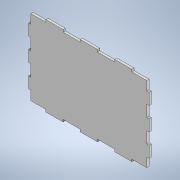
# Autodesk Inventor part: back
Saved by Autodesk Inventor 2020 (Build 240168000, 168)
## iProperties
Created: 2020-02-22
Part Number: back
Material: Generic
Document SubType Name: Modeling
Designer: udvarhelyi
Density: 1 g/cm^3
Appearance: Default
Author: udvarhelyi
Autodesk Inventor part; units mm, degrees
ref_plane "YZ Plane" through (0, 0, 0) normal (1, 0, 0) x (0, 1, 0)
ref_plane "XZ Plane" through (0, 0, 0) normal (0, 1, 0) x (-1, 0, 0)
ref_plane "XY Plane" through (0, 0, 0) normal (0, 0, 1) x (1, 0, 0)
sketch "Sketch1" plane through (0, 0, 0) normal (0, 0, 1) x (1, 0, 0)
  line L0 (-79, 15) -> (-76, 15)
  line L1 (-76, 30) -> (-79, 30)
  line L2 (-79, 45) -> (-76, 45)
  line L3 (-76, 60) -> (-79, 60)
  line L4 (-79, 75) -> (-76, 75)
  line L5 (-76, 90) -> (-79, 90)
  line L6 (76, 15) -> (79, 15)
  line L7 (76, 30) -> (79, 30)
  line L8 (79, 45) -> (76, 45)
  line L9 (76, 60) -> (79, 60)
  line L10 (79, 75) -> (76, 75)
  line L11 (79, 90) -> (76, 90)
  line L12 (-56.4286, 0) -> (-56.4286, 3)
  line L13 (-33.8571, 3) -> (-33.8571, 0)
  line L14 (-11.2857, 0) -> (-11.2857, 3)
  line L15 (11.2857, 0) -> (11.2857, 3)
  line L16 (33.8571, 0) -> (33.8571, 3)
  line L17 (56.4286, 0) -> (56.4286, 3)
  line L18 (-56.4286, 102) -> (-56.4286, 105)
  line L19 (-33.8571, 102) -> (-33.8571, 105)
  line L20 (-11.2857, 102) -> (-11.2857, 105)
  line L21 (11.2857, 102) -> (11.2857, 105)
  line L22 (33.8571, 102) -> (33.8571, 105)
  line L23 (56.4286, 102) -> (56.4286, 105)
  line L24 (-56.4286, 3) -> (-76, 3)
  line L25 (-76, 3) -> (-76, 15)
  line L26 (-76, 30) -> (-76, 45)
  line L27 (-76, 60) -> (-76, 75)
  line L28 (-76, 90) -> (-76, 102)
  line L29 (-76, 102) -> (-56.4286, 102)
  line L30 (-33.8571, 102) -> (-11.2857, 102)
  line L31 (11.2857, 102) -> (33.8571, 102)
  line L32 (56.4286, 102) -> (76, 102)
  line L33 (-11.2857, 3) -> (-33.8571, 3)
  line L34 (76, 3) -> (56.4286, 3)
  line L35 (33.8571, 3) -> (11.2857, 3)
  line L36 (-79, 75) -> (-79, 90)
  line L37 (-79, 15) -> (-79, 30)
  line L38 (-79, 45) -> (-79, 60)
  line L39 (-33.8571, 0) -> (-56.4286, 0)
  line L40 (56.4286, 0) -> (33.8571, 0)
  line L41 (11.2857, 0) -> (-11.2857, 0)
  line L42 (-56.4286, 105) -> (-33.8571, 105)
  line L43 (-11.2857, 105) -> (11.2857, 105)
  line L44 (33.8571, 105) -> (56.4286, 105)
  line L45 (79, 30) -> (79, 15)
  line L46 (79, 90) -> (79, 75)
  line L47 (79, 60) -> (79, 45)
  line L48 (76, 102) -> (76, 90)
  line L49 (76, 75) -> (76, 60)
  line L50 (76, 45) -> (76, 30)
  line L51 (76, 15) -> (76, 3)
  point P0 (0, 0)
  dimension "d1" = 158
  dimension "d5" = 22.5714
  dimension "d6" = 79
  dimension "d7" = 45.1429
  dimension "d8" = 67.7143
  dimension "d9" = 90.2857
  dimension "d10" = 112.8571
  dimension "d11" = 135.4286
  dimension "d12" = 105
  dimension "d13" = 15
  dimension "d14" = 0
  dimension "d15" = 3
  dimension "d16" = 30
  dimension "d17" = 45
  dimension "d18" = 60
  dimension "d19" = 75
  dimension "d20" = 90
  dimension "d21" = 99
  dimension "d22" = 3
  dimension "d23" = 3
  constraints: 104 end point, 79 perpendicular, 53 parallel, 21 collinear, 18 point on line, 3 horizontal
  measures "d1" distance of L5.end L11.start
  measures "d5" distance from line of L17.start L45
  measures "d6" distance from line of L46 point (0, 0)
  measures "d7" distance from line of L45 L16.start
  measures "d8" distance from line of L45 L15.end
  measures "d9" distance from line of L45 L14.start
  measures "d10" distance from line of L45 L13.end
  measures "d11" distance from line of L45 L12.start
  measures "d12" distance from line of L43 point (0, 0)
  measures "d13" distance from line of L0.start L39
  measures "d14" distance from line of point (0, 0) L39
  measures "d15" distance of L12.start L12.end
  measures "d16" distance from line of L39 L1.end
  measures "d17" distance from line of L39 L2.end
  measures "d18" distance from line of L39 L3.end
  measures "d19" distance from line of L39 L4.end
  measures "d20" distance from line of L39 L5.end
  measures "d21" distance between parallel lines of L24 L29
  measures "d22" distance of L11.start L11.end
  measures "d23" distance of L5.start L5.end
extrude "Extrusion1" add sketch "Sketch1" along normal blind 3
equation "\"d1\" = shelfWs"
equation "\"d5\" = 0.142857 * shelfWs - tol"
equation "\"d6\" = 0.5 * shelfWs"
equation "\"d7\" = 0.285714 * shelfWs + tol"
equation "\"d8\" = 0.428571 * shelfWs - tol"
equation "\"d9\" = 0.571429 * shelfWs + tol"
equation "\"d10\" = 0.714286 * shelfWs - tol"
equation "\"d11\" = 0.857143 * shelfWs + tol"
equation "\"d12\" = shelfD"
equation "\"d13\" = 0.142857 * shelfD - tol"
equation "\"d15\" = tt"
equation "\"d16\" = 0.285714 * shelfD + tol"
equation "\"d17\" = 0.428571 * shelfD - tol"
equation "\"d18\" = 0.571429 * shelfD + tol"
equation "\"d19\" = 0.714286 * shelfD - tol"
equation "\"d20\" = 0.857143 * shelfD + tol"
equation "\"d21\" = -2 * tt + shelfD"
equation "\"d22\" = tt"
equation "\"d23\" = tt"
equation "\"d24\" = tt"
equation "\"d0\" = 0.5 * shelfWs"
equation "\"tt\" = 3"
equation "\"tol\" = 0"
equation "\"d2\" = shelfD"
equation "\"d4\" = tt"
equation "\"tiroir\" = 1"
equation "\"nHoles\" = 4"
equation "\"shelfH\" = 35"
equation "\"shelfWs\" = 158"
equation "\"shelfD\" = 105"
body "Solid1"
